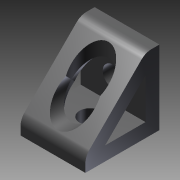
# Autodesk Inventor part: 4132
Saved by Autodesk Inventor 2016 (Build 200138000, 138)
## iProperties
Category: PARTsolutions
Company: 8020
Created: 2016-04-09
Part Number: 4132
Catalog Web Link: www.cadenas.de
Description: 4132, 4332-Joining Plates - 2 Hole Inside Gusset Corner Bracket
Vendor: 8020
Document SubType Name: Modeling
Designer: psAdmin
Manufacturer: 8020
Mass: 6.04683 g
Surface Area: 35.8011 cm^2
Volume: 6.04683 cm^3
Density: 1 g/cm^3
Material: Generic
Appearance: PSOLRGB-175-175-175
PSOL_IDENT_0: {$CADENAS_DATA\23d-libs\8020\inch\joining_plates\4132.prj},145 {VTYP=3D},{NB=4132},{LINA=4132},{NN=4
PSOL_IDENT_1: 132, 4332},{DATE=22.08.2012},{GEOMDATE=29.11.2011 00:00:00},{VERSION=},{LINEID=10},{LINESUBID=-1},{W
PSOL_IDENT_2: BVAR=}  {NB=4132},{LINA=4132},{KT=DUMMY},{PN=4132},{A=0.875},{B=1.000},{C=1.000},{E=0.188},{F=0.281}
PSOL_IDENT_3: ,{W=.041},{A1=0.4375},{C2=0.500},{D1=0.188},{C3=0.500}
NN: 4132, 4332
NT: Joining Plates - 2 Hole Inside Gusset Corner Bracket
NB: 4132
NBSYN: $PN.
LINA: 4132
PN: 4132
A: 0.875
B: 1.000
C: 1.000
W: .041
SUPPLIER: 8020
ARTICLENO: 4132
BOMINFO: 4132
CREATOR: CADENAS GmbH
Title: 4132
Author: Cadenas PARTsolutions
Comments: Joining Plates - 2 Hole Inside Gusset Corner Bracket
Autodesk Inventor part; units mm, degrees
ref_plane "YZ Plane" through (0, 0, 0) normal (1, 0, 0) x (0, 1, 0)
ref_plane "XZ Plane" through (0, 0, 0) normal (0, 1, 0) x (-1, 0, 0)
ref_plane "XY Plane" through (0, 0, 0) normal (0, 0, 1) x (1, 0, 0)
sketch "Sketch_1" plane through (0, 0, 0) normal (1, 0, 0) x (0, 1, 0)
  line L0 (2.7972, 25.4) -> (0, 25.4)
  line L1 (0, 25.4) -> (0, 0)
  line L2 (0, 0) -> (25.4, 0)
  line L3 (25.4, 0) -> (25.4, 2.7972)
  arc A0 (25.4, 2.7972) -> (24.0014, 6.1738) centre (20.6248, 2.7972) ccw
  line L4 (24.0014, 6.1738) -> (6.1738, 24.0014)
  arc A1 (6.1738, 24.0014) -> (2.7972, 25.4) centre (2.7972, 20.6248) ccw
  line L5 (4.7752, 18.6468) -> (4.7752, 4.7752)
  line L6 (4.7752, 4.7752) -> (18.6468, 4.7752)
  line L7 (18.6468, 4.7752) -> (4.7752, 18.6468)
  constraints: 16 end point, 4 point on circle, 2 centre point
extrude "Extrusion1" add sketch "Sketch_1" along normal mid plane 22.225
sketch "Sketch2" plane through (-11.1125, 0, 25.4) normal (0, -1, 0) x (1, 0, 0)
  point P0 (11.1125, -12.7)
hole "Hole1" at (0, 0, 12.7) direction (0, 1, 0) diameter 7.1374 depth 4.7752
sketch "Sketch3" plane through (11.1125, 0, 0) normal (0, 0, -1) x (-1, 0, 0)
  point P0 (11.1125, 12.7)
hole "Hole2" at (0, 12.7, 0) direction (0, 0, 1) diameter 7.1374 depth 4.7752
sketch "Sketch_4" plane through (0, 0, 25.4) normal (0, 0, 1) x (1, 0, 0)
  circle A0 centre (0, 12.7) radius 6.35
  constraints: 1 centre point
extrude "Extrusion2" cut sketch "Sketch_4" against normal blind 20.6248
sketch "Sketch_5" plane through (0, 25.4, 0) normal (0, 1, 0) x (1, 0, 0)
  circle A0 centre (0, -12.7) radius 6.35
  constraints: 1 centre point
extrude "Extrusion3" cut sketch "Sketch_5" against normal blind 20.6248
body "Solid1"
